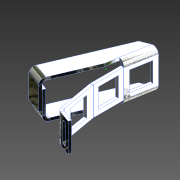
# Autodesk Inventor part: ThumbPlate
Saved by Autodesk Inventor 2018 (Build 220112000, 112)
## iProperties
Created: 2018-05-27
Part Number: ThumbPlate
Material: アルミニウム 6061
Document SubType Name: Sheet Metal
Designer: NaMACHAN
Mass: 3.96198 g
Surface Area: 20.72 cm^2
Volume: 1.4674 cm^3
Density: 2.7 g/cm^3
Sheet Metal Rule: Al2
Appearance: アルミニウム - フラット
Author: NaMACHAN
Autodesk Inventor part; units mm, degrees
ref_plane "YZ Plane" through (0, 0, 0) normal (1, 0, 0) x (0, 1, 0)
ref_plane "XZ Plane" through (0, 0, 0) normal (0, 1, 0) x (-1, 0, 0)
ref_plane "XY Plane" through (0, 0, 0) normal (0, 0, 1) x (1, 0, 0)
sketch "スケッチ1" plane through (0, 0, 0) normal (1, 0, 0) x (0, 1, 0)
  line L0 (-10.5, -10) -> (10.5, -10)
  line L1 (10.5, -10) -> (10.5, 10)
  line L2 (10.5, 10) -> (-10.5, 10)
  line L3 (-10.5, 10) -> (-10.5, -10)
  line L4 (-10.5, -10) -> (10.5, 10) construction
  line L5 (10.5, -10) -> (-10.5, 10) construction
  point P0 (0, 0)
  dimension "d0" = 21
  dimension "d1" = 20
  measures "d0" distance of L2.end L1.end
  measures "d1" distance of L1.end L0.end
extrude "プレート1" add sketch "スケッチ1" along normal blind 2
sketch "スケッチ3" plane through (2.0304, -10.8473, -10) normal (-0.9848078, -0.1736482, 0) x (0.1736482, -0.9848078, 0)
  line L0 (0, 20) -> (0, 0)
  line L1 (0, 0) -> (24.65, 0)
  line L2 (24.65, 0) -> (24.65, 20)
  line L3 (24.65, 20) -> (0, 20)
  constraints: 6 end point, 1 horizontal, 1 perpendicular, 1 vertical
edge flange "フランジ2" height 25 angle 10 thickness 2 bend radius 2 thickness toward (-0.9848078, -0.1736482, 0) relief tear relief width 2 relief depth 1 edges at (2, -10.5, 0) wall of the first edge with corners at (2.0304, -10.8473, 10) (2.0304, -10.8473, -10) (6.3108, -35.1229, -10) (6.3108, -35.1229, 10)
bend "曲げ2"
corner "コーナー2"
sketch "スケッチ5" plane through (2, 0, 0) normal (1, 0, 0) x (0, 0, -1)
  line L0 (7, -7) -> (-7, -7)
  line L1 (-7, -7) -> (-7, 7)
  line L2 (-7, 7) -> (7, 7)
  line L3 (7, 7) -> (7, -7)
  line L4 (7, -7) -> (-7, 7) construction
  line L5 (-7, -7) -> (7, 7) construction
  point P0 (0, 0)
  dimension "d27" = 14
  dimension "d28" = 14
  constraints: 12 end point, 2 midpoint, 2 parallel, 1 horizontal, 1 perpendicular
  measures "d27" distance of L1.end L2.end
  measures "d28" distance of L0.end L1.end
extrude "押し出し2" cut sketch "スケッチ5" against normal blind 10
sketch "スケッチ6" plane through (6.3108, -35.1229, 10) normal (0.9848078, 0.1736482, 0) x (0, 0, -1)
  line L0 (17, 5.325) -> (3, 5.325)
  line L1 (3, 5.325) -> (3, 19.325)
  line L2 (3, 19.325) -> (17, 19.325)
  line L3 (17, 19.325) -> (17, 5.325)
  line L4 (17, 5.325) -> (3, 19.325) construction
  line L5 (3, 5.325) -> (17, 19.325) construction
  line L6 (20, 0) -> (20, 24.65) projected
  line L7 (17, 28.4442) -> (3, 28.4442) projected
  point P0 (10, 35.6851)
  point P1 (10, 12.325)
  point P2 (10, 12.325)
  point P3 (20, 12.325)
  point P4 (10, 12.325)
  point P5 (10, 28.4442)
  dimension "d31" = 14
  dimension "d32" = 14
  constraints: 12 end point, 6 midpoint, 2 parallel, 1 horizontal, 1 horizontal alignment, 1 perpendicular, 1 vertical alignment
  measures "d31" distance of L1.end L2.end
  measures "d32" distance of L0.end L1.end
extrude "押し出し3" cut sketch "スケッチ6" against normal blind 10
sketch "スケッチ7" plane through (7.5964, -36.6549, 10) normal (-0.3420201, -0.9396926, 0) x (-0.9396926, 0.3420201, 0)
  line L0 (0, -20) -> (0, 0)
  line L1 (0, 0) -> (-8.8453, 0)
  line L2 (-8.8453, 0) -> (-8.8453, -20)
  line L3 (-8.8453, -20) -> (0, -20)
  constraints: 6 end point, 1 horizontal, 1 perpendicular, 1 vertical
edge flange "フランジ3" height 10 angle -60 thickness 2 bend radius 2 thickness toward (-0.3420201, -0.9396926, 0) relief tear relief width 2 relief depth 1 edges at (4.3412, -35.4701, 0) wall of the first edge with corners at (7.5964, -36.6549, -10) (7.5964, -36.6549, 10) (15.9083, -39.6802, 10) (15.9083, -39.6802, -10)
bend "曲げ3"
corner "コーナー3"
sketch "スケッチ8" plane through (15.9083, -39.6802, 10) normal (0.3420201, 0.9396926, 0) x (0.9396926, -0.3420201, 0)
  line L0 (-5.9226, 4) -> (-5.9226, 16)
  arc A0 (-2.9226, 16) -> (-5.9226, 16) centre (-4.4226, 16) ccw
  line L1 (-2.9226, 16) -> (-2.9226, 4)
  arc A1 (-5.9226, 4) -> (-2.9226, 4) centre (-4.4226, 4) ccw
  line L2 (-8.8453, 20) -> (0, 20) projected
  line L3 (0, 0) -> (-8.8453, 0) projected
  point P0 (-28.5203, 10)
  point P1 (-4.4226, 20)
  dimension "d45" = 4
  dimension "d46" = 4
  dimension "d47" = 1.5
  constraints: 4 end point, 4 point on circle, 4 tangent, 2 centre point, 1 midpoint, 1 parallel, 1 vertical, 1 vertical alignment
  measures "d45" distance from line of L2 A0.centre
  measures "d46" distance from line of L3 A1.centre
  measures "d47" radius of A1
extrude "押し出し4" cut sketch "スケッチ8" against normal blind 10
sketch "スケッチ25" plane through (-2, 12.5, -10) normal (0, 1, 0) x (-1, 0, 0)
  line L0 (0, 20) -> (0, 0)
  line L1 (0, 0) -> (8, 0)
  line L2 (8, 0) -> (8, 20)
  line L3 (8, 20) -> (0, 20)
  constraints: 6 end point, 1 horizontal, 1 perpendicular, 1 vertical
edge flange "フランジ12" height 10 angle 90 thickness 2 bend radius 2 thickness toward (0, 1, 0) relief tear relief width 2 relief depth 1 edges at (0, 10.5, 0) wall of the first edge with corners at (-2, 12.5, 10) (-2, 12.5, -10) (-10, 12.5, -10) (-10, 12.5, 10)
bend "曲げ21"
corner "コーナー12"
sketch "スケッチ26" plane through (-11.9696, 10.8473, -10) normal (-0.9848078, 0.1736482, 0) x (-0.1736482, -0.9848078, 0)
  line L0 (0, 20) -> (0, 0)
  line L1 (0, 0) -> (37.0268, 0)
  line L2 (37.0268, 0) -> (37.0268, 20)
  line L3 (37.0268, 20) -> (0, 20)
  constraints: 6 end point, 1 horizontal, 1 perpendicular, 1 vertical
edge flange "フランジ13" height 38.705 angle 80 thickness 2 bend radius 2 thickness toward (-0.9848078, 0.1736482, 0) relief tear relief width 2 relief depth 1 edges at (-10, 12.5, 0) wall of the first edge with corners at (-11.9696, 10.8473, 10) (-11.9696, 10.8473, -10) (-18.3993, -25.617, -10) (-18.3993, -25.617, 10)
bend "曲げ22"
corner "コーナー13"
sketch "スケッチ27" plane through (-17.1137, -27.8437, -10) normal (-0.3420201, -0.9396926, 0) x (0.9396926, -0.3420201, 0)
  line L0 (0, 20) -> (0, 0)
  line L1 (0, 0) -> (8.3218, 0)
  line L2 (8.3218, 0) -> (8.3218, 20)
  line L3 (8.3218, 20) -> (0, 20)
  constraints: 6 end point, 1 horizontal, 1 perpendicular, 1 vertical
edge flange "フランジ14" height 10 angle 80 thickness 2 bend radius 2 thickness toward (-0.3420201, -0.9396926, 0) relief tear relief width 2 relief depth 1 edges at (-18.3993, -25.617, 0) wall of the first edge with corners at (-17.1137, -27.8437, 10) (-17.1137, -27.8437, -10) (-9.2937, -30.6899, -10) (-9.2937, -30.6899, 10)
bend "曲げ23"
corner "コーナー14"
sketch "スケッチ28" plane through (-9.2937, -30.6899, 10) normal (0.3420201, 0.9396926, 0) x (0.9396926, -0.3420201, 0)
  line L0 (-5.6609, 4) -> (-5.6609, 16)
  arc A0 (-2.6609, 16) -> (-5.6609, 16) centre (-4.1609, 16) ccw
  line L1 (-2.6609, 16) -> (-2.6609, 4)
  line L2 (-2.2781, 3) -> (-2.2781, 17) projected
  arc A1 (-5.6609, 4) -> (-2.6609, 4) centre (-4.1609, 4) ccw
  line L3 (0, 0) -> (-8.3218, 0) projected
  line L4 (0, 20) -> (-8.3218, 20) projected
  point P0 (-1.7633, 10)
  point P1 (-4.1609, 20)
  dimension "d224" = 4
  dimension "d225" = 4
  dimension "d226" = 1.5
  constraints: 4 end point, 4 point on circle, 2 centre point, 2 parallel, 2 tangent, 2 vertical alignment, 1 horizontal alignment, 1 midpoint
  measures "d224" distance from line of L3 A1.centre
  measures "d225" distance from line of L4 A0.centre
  measures "d226" radius of A1
extrude "押し出し6" cut sketch "スケッチ28" against normal blind 10
equation "\"d2\" = Thickness"
equation "\"d13\" = BendReliefWidth"
equation "\"d14\" = BendReliefDepth"
equation "\"d15\" = MinimumRemnant"
equation "\"d16\" = TransitionRadius"
equation "\"d19\" = BendRadius"
equation "\"d20\" = CornerReliefSize"
equation "\"d21\" = GapSize"
equation "\"d22\" = JacobiRadiusSize"
equation "\"d35\" = BendReliefWidth"
equation "\"d36\" = BendReliefDepth"
equation "\"d37\" = MinimumRemnant"
equation "\"d38\" = TransitionRadius"
equation "\"d41\" = BendRadius"
equation "\"d42\" = CornerReliefSize"
equation "\"d43\" = GapSize"
equation "\"d44\" = JacobiRadiusSize"
equation "\"d194\" = BendReliefWidth"
equation "\"d195\" = BendReliefDepth"
equation "\"d196\" = MinimumRemnant"
equation "\"d197\" = TransitionRadius"
equation "\"d200\" = BendRadius"
equation "\"d201\" = CornerReliefSize"
equation "\"d202\" = GapSize"
equation "\"d203\" = JacobiRadiusSize"
equation "\"d204\" = BendReliefWidth"
equation "\"d205\" = BendReliefDepth"
equation "\"d206\" = MinimumRemnant"
equation "\"d207\" = TransitionRadius"
equation "\"d210\" = BendRadius"
equation "\"d211\" = CornerReliefSize"
equation "\"d212\" = GapSize"
equation "\"d213\" = JacobiRadiusSize"
equation "\"d214\" = BendReliefWidth"
equation "\"d215\" = BendReliefDepth"
equation "\"d216\" = MinimumRemnant"
equation "\"d217\" = TransitionRadius"
equation "\"d220\" = BendRadius"
equation "\"d221\" = CornerReliefSize"
equation "\"d222\" = GapSize"
equation "\"d223\" = JacobiRadiusSize"
equation "\"BendRadius\" = Thickness"
equation "\"BendReliefWidth\" = Thickness"
equation "\"BendReliefDepth\" = 0.5 * Thickness"
equation "\"CornerReliefSize\" = 4 * Thickness"
equation "\"MinimumRemnant\" = 2 * Thickness"
equation "\"TransitionRadius\" = BendRadius"
equation "\"JacobiRadiusSize\" = BendRadius"
equation "\"GapSize\" = Thickness"
equation "\"Thickness\" = 2"
